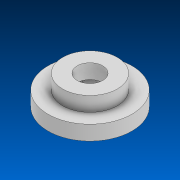
# Autodesk Inventor part: Standoff Connector
Saved by Autodesk Inventor 2022 (Build 260153000, 153)
## iProperties
Created: 2022-04-05
Part Number: Standoff Connector
Material: Generic
Document SubType Name: Modeling
Designer: score_nygvs6w
Density: 1 g/cm^3
Appearance: Default
Author: score_nygvs6w
Autodesk Inventor part; units mm, degrees
ref_plane "YZ Plane" through (0, 0, 0) normal (1, 0, 0) x (0, 1, 0)
ref_plane "XZ Plane" through (0, 0, 0) normal (0, 1, 0) x (-1, 0, 0)
ref_plane "XY Plane" through (0, 0, 0) normal (0, 0, 1) x (1, 0, 0)
sketch "Sketch1" plane through (0, 0, 0) normal (0, 0, 1) x (1, 0, 0)
  line L0 (2.2225, 0) -> (2.2225, 2.54)
  line L1 (2.2225, 2.54) -> (4.7625, 2.54)
  line L2 (4.7625, 2.54) -> (4.7625, 0)
  line L3 (4.7625, 0) -> (7.3025, 0)
  line L4 (7.3025, 0) -> (7.3025, -2.54)
  line L5 (7.3025, -2.54) -> (3.175, -2.54)
  line L6 (3.175, -2.54) -> (3.175, 0)
  line L7 (3.175, 0) -> (2.2225, 0)
  line L8 (-5.2705, 0) -> (9.398, 0) projected
  line L9 (0, -3.556) -> (0, 3.556) projected
  point P0 (0, 0)
  dimension "d0" = 2.2225
  dimension "d1" = 4.7625
  dimension "d2" = 2.54
  dimension "d3" = 2.54
  dimension "d4" = 2.54
  dimension "d7" = 3.175
  constraints: 16 end point, 6 perpendicular, 1 collinear, 1 parallel, 1 point on line, 1 vertical
  measures "d0" distance from line of point (0, 0) L0
  measures "d1" distance from line of point (0, 0) L2
  measures "d2" distance between parallel lines of L3 L5
  measures "d3" distance between parallel lines of L7 L1
  measures "d4" distance between parallel lines of L2 L4
  measures "d7" distance from line of point (0, 0) L6
revolve "Revolution1" add sketch "Sketch1" angle 360 about axis through (0, -10, 0) along (0, 1, 0)
sketch "Sketch2" plane through (0, 0, 0) normal (0, -1, 0) x (1, 0, 0)
  line L0 (0, 3.6662) -> (3.175, 1.8331)
  line L1 (3.175, 1.8331) -> (3.175, -1.8331)
  line L2 (3.175, -1.8331) -> (0, -3.6662)
  line L3 (0, -3.6662) -> (-3.175, -1.8331)
  line L4 (-3.175, -1.8331) -> (-3.175, 1.8331)
  line L5 (-3.175, 1.8331) -> (0, 3.6662)
  point P0 (0, 0)
  point P1 (0, 0)
  dimension "d8" = 6.35
  constraints: 12 end point, 1 coincident, 1 vertical, 13 other
  measures "d8" distance between parallel lines of L4 L1
extrude "Extrusion1" cut sketch "Sketch2" along normal blind 25.4
body "Solid1"
